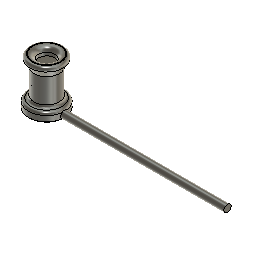
lung_intubate (Autodesk Fusion 360 design; units mm, degrees)
Autodesk Fusion 360 part; units mm, degrees
sketch "Sketch1" plane through (0, 0, 0) normal (0, 0, 1) x (1, 0, 0)
  circle A0 centre (0, 0) radius 10
  dimension "d1" = 20
  constraint coincident A0.centre origin
  measures "d1" diameter of A0
extrude "Extrude1" add sketch "Sketch1" along normal blind 5
sketch "Sketch2" plane through (0, 0, 5) normal (0, 0, 1) x (-1, 0, 0)
  circle A0 centre (0, 0) radius 10
  circle A1 centre (0, 0) radius 7
  dimension "d4" = 14
  constraint concentric A0 A1
  measures "d4" diameter of A1
extrude "Extrude2" add sketch "Sketch2" along normal blind 15 contours A1
sketch "Sketch3" plane through (0, 0, 0) normal (1, 0, 0) x (0, 1, 0)
  circle A0 centre (0, 2) radius 2
  dimension "d7" = 4
  measures "d7" diameter of A0
extrude "Extrude3" cut sketch "Sketch3" along normal blind 17
extrude "Extrude4" add 1 faces at (0, 0.6381, 2.1226) along direction (1, 0, 0) blind 100
fillet "Fillet1" radius 1.5 1 faces at (8.9367, -0.8446, 5)
extrude "Extrude5" add 1 faces at (-1.3617, -1.5871, 20) along direction (0, 0, 1) blind 6 draft 30
fillet "Fillet2" radius 1.5 1 faces at (2.7119, 3.4006, 26)
fillet "Fillet3" radius 0.5 1 edges at (-9.3233, -3.6162, 0)
sketch "Sketch4" plane through (0, 0, 26) normal (0, 0, 1) x (-1, 0, 0)
  circle A0 centre (0, 0) radius 7.866
  circle A1 centre (0, 0) radius 5
  dimension "d20" = 10
  constraint concentric A0 A1
  measures "d20" diameter of A1
extrude "Extrude6" cut sketch "Sketch4" against normal blind 4 draft -10 contours A1
fillet "Fillet4" radius 3 1 edges at (4.6616, -1.8081, 26)
sketch "Sketch5" plane through (0, 0, 0) normal (0, 0, 1) x (1, 0, 0)
  circle A0 centre (0, 0) radius 6.5
  dimension "d25" = 13
  constraint coincident A0.centre origin
  measures "d25" diameter of A0
extrude "Extrude7" cut sketch "Sketch5" along normal blind 13
fillet "Fillet5" radius 1.5 1 edges at (-6.0601, -2.3505, 0)
